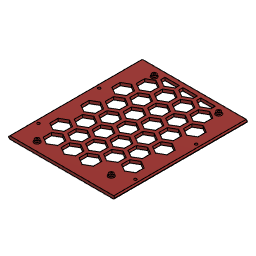
MCU Tray - BTT Manta M8P (Autodesk Fusion 360 design; units mm, degrees)
Autodesk Fusion 360 part; units mm, degrees
note: some values were not read from the file. Chosen so that the rebuilt part matches the saved one: a direction.
imported_body "Derived Base Feature2" makes body 1
imported_body "Derived Base Feature1" makes body 2
sketch "Base Profile" plane through (0, 0, 0) normal (0, 1, 0) x (1, 0, 0)
  line L0 (72.5, 2) -> (-72.5, 2)
  line L1 (-72.5, 2) -> (-72.5, -2) construction
  line L2 (-72.5, -2) -> (72.5, -2)
  line L3 (72.5, -2) -> (72.5, 2) construction
  line L4 (72.5, 2) -> (-72.5, -2) construction
  line L5 (-72.5, 2) -> (72.5, -2) construction
  line L6 (-72.5, 0) -> (-74.3, 0) construction
  line L7 (-72.5, -2) -> (-74.3, -0.2)
  line L8 (-74.3, 0.2) -> (-72.5, 2)
  line L9 (-74.3, -0.2) -> (-74.3, 0)
  line L10 (-74.3, 0) -> (-74.3, 0.2)
  line L11 (0, 0) -> (0, -2) construction
  line L12 (72.5, -2) -> (74.3, -0.2)
  line L13 (74.3, -0.2) -> (74.3, 0)
  line L14 (74.3, 0) -> (74.3, 0.2)
  line L15 (74.3, 0.2) -> (72.5, 2)
  dimension "d1" = 145
  dimension "d2" = 4
  dimension "d3" = 0.2
  constraint horizontal L0
  constraint perpendicular L0 L1
  constraint parallel L0 L2
  constraint parallel L1 L3
  constraint coincident L4 L11.start
  constraint coincident L5 L11.start
  constraint coincident L11.start origin
  constraint midpoint L1 L6.start
  constraint perpendicular L1 L6
  constraint coincident L5 L0.end
  constraint coincident L0 L1.start
  constraint perpendicular L6 L9
  constraint perpendicular L6 L10
  constraint midpoint L2 L11.end
  constraint symmetric L1.end L11 L2.end
  constraint symmetric L0.end L11 L0.start
  constraint symmetric L7.end L11 L12.end
  constraint symmetric L6.end L11 L13.end
  constraint symmetric L8.start L11 L14.end
  measures "d1" distance of L1.end L2.end
  measures "d2" distance of L0.end L1.end
  measures "d3" distance of L7.end L6.end
extrude "Extrude1" add sketch "Base Profile" along normal blind 190 and the other way blind 15 separate body makes body 3
sketch "M3 Mount Holes" plane through (0, 0, 2) normal (0, 0, 1) x (-1, 0, 0)
  line L0 (72.5, 15) -> (-72.5, 15)
  line L1 (-72.5, 15) -> (-72.5, -190)
  line L2 (-72.5, -190) -> (72.5, -190)
  line L3 (72.5, -190) -> (72.5, 15)
  line L4 (0, 0) -> (0, -28.0831) construction
  circle A0 centre (-67.6414, -20) radius 1.8
  line L5 (72.6414, -59.8458) -> (72.6414, 0.0002) construction
  circle A1 centre (67.6414, -20) radius 1.8
  line L6 (72.5, -190) -> (72.5, 15)
  line L7 (72.6414, 0.0002) -> (78.5, 0.0002)
  line L8 (67.6414, -20) -> (72.6414, -20) construction
  line L9 (72.6414, -20) -> (72.6414, 0.0002) construction
  line L10 (67.6414, -20) -> (67.6414, -105) construction
  circle A2 centre (67.6414, -105) radius 1.8
  circle A3 centre (-67.6414, -105) radius 1.8
  dimension "d16" = 3.6
  dimension "d17" = 85
  dimension "d18" = 3.6
  dimension "d42" = 5
  dimension "d43" = 35
  constraint coincident L4.start origin
  constraint vertical L4
  constraint symmetric L4 A0 A1
  constraint horizontal L8
  constraint vertical L9
  constraint coincident L5.end L7.start
  constraint coincident A1.centre L8.start
  constraint perpendicular L8 L10
  constraint coincident L10.end A2.centre
  constraint symmetric L4 A2 A3
  measures "d16" diameter of A1
  measures "d17" distance of A1.centre L10.end
  measures "d18" diameter of A2
  measures "d42" distance of A1.centre L8.end
  measures "d43" distance of L0 A1.centre
sketch "M4 Mount Holes" plane through (0, 0, 2) normal (0, 0, 1) x (-1, 0, 0)
  line L0 (-72.5, 15) -> (-72.5, -190)
  line L1 (-72.5, -190) -> (72.5, -190)
  line L2 (72.5, -190) -> (72.5, 15)
  line L3 (72.5, 15) -> (-72.5, 15)
  circle A0 centre (-67.6414, -20) radius 1.8 construction
  circle A1 centre (-67.6414, -20) radius 2.3
  line L4 (-67.6414, -20) -> (-67.6414, -105) construction
  circle A2 centre (-67.6414, -105) radius 2.3
  line L5 (0, 0) -> (0, -39.5368) construction
  circle A3 centre (67.6414, -105) radius 2.3
  circle A4 centre (67.6414, -20) radius 2.3
  dimension "d37" = 4.6
  dimension "d38" = 85
  dimension "d39" = 4.6
  constraint concentric A0 A1
  constraint coincident A0.centre A1.centre
  constraint parallel L0 L4
  constraint coincident L4.end A2.centre
  constraint coincident L5.start origin
  constraint vertical L5
  constraint symmetric A1 L5 A4
  constraint symmetric A2 L5 A3
  measures "d37" diameter of A1
  measures "d38" distance of A0.centre L4.end
  measures "d39" diameter of A2
extrude "Extrude2" cut sketch "M3 Mount Holes" against normal up to surface (4 mm away) contours A0 | A1 | A2 | A3 bodies 3
extrude "Extrude5" [suppressed]
extrude "Extrude3" cut 1 faces at (24.1667, 190, 0.6667) along direction (0, -1, 0) blind 40.154 on bodies 3 bodies 3
delete_body "RemoveBody1" bodies 2
delete_body "RemoveBody2" bodies 1
move_face "OffsetFaces2" offset 20 1 faces at (24.1667, 149.846, 0.6667) on bodies 3
sketch "Vent Holes" plane through (0, 0, 2) normal (0, 0, 1) x (-1, 0, 0)
  line L0 (-72.5, -169.846) -> (72.5, -169.846)
  line L1 (72.5, -169.846) -> (72.5, 15)
  line L2 (72.5, 15) -> (-72.5, 15)
  line L3 (-72.5, 15) -> (-72.5, -169.846)
  line L4 (0, 15) -> (0, -169.846) construction
  line L5 (10, -71.6495) -> (0, -65.876)
  line L6 (0, -65.876) -> (-10, -71.6495)
  line L7 (-10, -71.6495) -> (-10, -83.1965)
  line L8 (-10, -83.1965) -> (0, -88.97)
  line L9 (0, -88.97) -> (10, -83.1965)
  line L10 (10, -83.1965) -> (10, -71.6495)
  line L11 (0, -77.423) -> (5, -86.0833) construction
  line L12 (0, -77.423) -> (-5, -86.0833) construction
  line L13 (-15, -28.3482) -> (-25, -22.5747)
  line L14 (-25, -22.5747) -> (-35, -28.3482)
  line L15 (-35, -28.3482) -> (-35, -39.8952)
  line L16 (-35, -39.8952) -> (-25, -45.6687)
  line L17 (-25, -45.6687) -> (-15, -39.8952)
  line L18 (-15, -39.8952) -> (-15, -28.3482)
  line L19 (-27.5, -6.6976) -> (-37.5, -0.9241)
  line L20 (-37.5, -0.9241) -> (-47.5, -6.6976)
  line L21 (-47.5, -6.6976) -> (-47.5, -18.2446)
  line L22 (-47.5, -18.2446) -> (-37.5, -24.0181)
  line L23 (-37.5, -24.0181) -> (-27.5, -18.2446)
  line L24 (-27.5, -18.2446) -> (-27.5, -6.6976)
  line L25 (-2.5, -49.9989) -> (-12.5, -44.2254)
  line L26 (-12.5, -44.2254) -> (-22.5, -49.9989)
  line L27 (-22.5, -49.9989) -> (-22.5, -61.5459)
  line L28 (-22.5, -61.5459) -> (-12.5, -67.3194)
  line L29 (-12.5, -67.3194) -> (-2.5, -61.5459)
  line L30 (-2.5, -61.5459) -> (-2.5, -49.9989)
  line L31 (22.5, -93.3001) -> (12.5, -87.5266)
  line L32 (12.5, -87.5266) -> (2.5, -93.3001)
  line L33 (2.5, -93.3001) -> (2.5, -104.8471)
  line L34 (2.5, -104.8471) -> (12.5, -110.6206)
  line L35 (12.5, -110.6206) -> (22.5, -104.8471)
  line L36 (22.5, -104.8471) -> (22.5, -93.3001)
  line L37 (35, -114.9508) -> (25, -109.1773)
  line L38 (25, -109.1773) -> (15, -114.9508)
  line L39 (15, -114.9508) -> (15, -126.4978)
  line L40 (15, -126.4978) -> (25, -132.2713)
  line L41 (25, -132.2713) -> (35, -126.4978)
  line L42 (35, -126.4978) -> (35, -114.9508)
  line L43 (47.5, -136.6014) -> (37.5, -130.8279)
  line L44 (37.5, -130.8279) -> (27.5, -136.6014)
  line L45 (27.5, -136.6014) -> (27.5, -148.1484)
  line L46 (27.5, -148.1484) -> (37.5, -153.9219)
  line L47 (37.5, -153.9219) -> (47.5, -148.1484)
  line L48 (47.5, -148.1484) -> (47.5, -136.6014)
  line L49 (12.5, -67.3194) -> (22.5, -61.5459)
  line L50 (22.5, -61.5459) -> (22.5, -49.9989)
  line L51 (22.5, -49.9989) -> (12.5, -44.2254)
  line L52 (12.5, -44.2254) -> (2.5, -49.9989)
  line L53 (2.5, -61.5459) -> (12.5, -67.3194)
  line L54 (2.5, -49.9989) -> (2.5, -61.5459)
  line L55 (-15, -71.6495) -> (-25, -65.876)
  line L56 (-25, -65.876) -> (-35, -71.6495)
  line L57 (-35, -71.6495) -> (-35, -83.1965)
  line L58 (-35, -83.1965) -> (-25, -88.97)
  line L59 (-15, -83.1965) -> (-15, -71.6495)
  line L60 (-25, -88.97) -> (-15, -83.1965)
  line L61 (-2.5, -6.6976) -> (-12.5, -0.9241)
  line L62 (-12.5, -0.9241) -> (-22.5, -6.6976)
  line L63 (-22.5, -6.6976) -> (-22.5, -18.2446)
  line L64 (-22.5, -18.2446) -> (-12.5, -24.0181)
  line L65 (-12.5, -24.0181) -> (-2.5, -18.2446)
  line L66 (-2.5, -18.2446) -> (-2.5, -6.6976)
  line L67 (-40, -28.3482) -> (-50, -22.5747)
  line L68 (-50, -22.5747) -> (-60, -28.3482)
  line L69 (-60, -28.3482) -> (-60, -39.8952)
  line L70 (-60, -39.8952) -> (-50, -45.6687)
  line L71 (-40, -39.8952) -> (-40, -28.3482)
  line L72 (-50, -45.6687) -> (-40, -39.8952)
  line L73 (10, -28.3482) -> (0, -22.5747)
  line L74 (0, -22.5747) -> (-10, -28.3482)
  line L75 (-10, -28.3482) -> (-10, -39.8952)
  line L76 (-10, -39.8952) -> (0, -45.6687)
  line L77 (0, -45.6687) -> (10, -39.8952)
  line L78 (10, -39.8952) -> (10, -28.3482)
  line L79 (-27.5, -49.9989) -> (-37.5, -44.2254)
  line L80 (-37.5, -44.2254) -> (-47.5, -49.9989)
  line L81 (-47.5, -49.9989) -> (-47.5, -61.5459)
  line L82 (-47.5, -61.5459) -> (-37.5, -67.3194)
  line L83 (-27.5, -61.5459) -> (-27.5, -49.9989)
  line L84 (-37.5, -67.3194) -> (-27.5, -61.5459)
  line L85 (35, -71.6495) -> (25, -65.876)
  line L86 (25, -65.876) -> (15, -71.6495)
  line L87 (15, -71.6495) -> (15, -83.1965)
  line L88 (15, -83.1965) -> (25, -88.97)
  line L89 (25, -88.97) -> (35, -83.1965)
  line L90 (35, -83.1965) -> (35, -71.6495)
  line L91 (-2.5, -93.3001) -> (-12.5, -87.5266)
  line L92 (-12.5, -87.5266) -> (-22.5, -93.3001)
  line L93 (-22.5, -93.3001) -> (-22.5, -104.8471)
  line L94 (-22.5, -104.8471) -> (-12.5, -110.6206)
  line L95 (-2.5, -104.8471) -> (-2.5, -93.3001)
  line L96 (-12.5, -110.6206) -> (-2.5, -104.8471)
  line L97 (47.5, -93.3001) -> (37.5, -87.5266)
  line L98 (37.5, -87.5266) -> (27.5, -93.3001)
  line L99 (27.5, -93.3001) -> (27.5, -104.8471)
  line L100 (27.5, -104.8471) -> (37.5, -110.6206)
  line L101 (37.5, -110.6206) -> (47.5, -104.8471)
  line L102 (47.5, -104.8471) -> (47.5, -93.3001)
  line L103 (10, -114.9508) -> (0, -109.1773)
  line L104 (0, -109.1773) -> (-10, -114.9508)
  line L105 (-10, -114.9508) -> (-10, -126.4978)
  line L106 (-10, -126.4978) -> (0, -132.2713)
  line L107 (10, -126.4978) -> (10, -114.9508)
  line L108 (0, -132.2713) -> (10, -126.4978)
  line L109 (60, -114.9508) -> (50, -109.1773)
  line L110 (50, -109.1773) -> (40, -114.9508)
  line L111 (40, -114.9508) -> (40, -126.4978)
  line L112 (40, -126.4978) -> (50, -132.2713)
  line L113 (50, -132.2713) -> (60, -126.4978)
  line L114 (60, -126.4978) -> (60, -114.9508)
  line L115 (22.5, -136.6014) -> (12.5, -130.8279)
  line L116 (12.5, -130.8279) -> (2.5, -136.6014)
  line L117 (2.5, -136.6014) -> (2.5, -148.1484)
  line L118 (2.5, -148.1484) -> (12.5, -153.9219)
  line L119 (22.5, -148.1484) -> (22.5, -136.6014)
  line L120 (12.5, -153.9219) -> (22.5, -148.1484)
  line L121 (-47.5, -55.7724) -> (-60, -55.7724) construction
  line L122 (-40, -71.6495) -> (-40, -83.1965)
  line L123 (-40, -83.1965) -> (-50, -88.97)
  line L124 (-50, -88.97) -> (-60, -83.1965)
  line L125 (-60, -83.1965) -> (-60, -71.6495)
  line L126 (-60, -71.6495) -> (-50, -65.876)
  line L127 (-50, -65.876) -> (-40, -71.6495)
  line L128 (47.5, -99.0736) -> (60, -99.0736) construction
  line L129 (40, -83.1965) -> (40, -71.6495)
  line L130 (40, -71.6495) -> (50, -65.876)
  line L131 (50, -65.876) -> (60, -71.6495)
  line L132 (60, -71.6495) -> (60, -83.1965)
  line L133 (60, -83.1965) -> (50, -88.97)
  line L134 (50, -88.97) -> (40, -83.1965)
  line L135 (-47.5, -104.8471) -> (-47.5, -93.3001)
  line L136 (-47.5, -93.3001) -> (-37.5, -87.5266)
  line L137 (-37.5, -87.5266) -> (-27.5, -93.3001)
  line L138 (-27.5, -93.3001) -> (-27.5, -104.8471)
  line L139 (-27.5, -104.8471) -> (-37.5, -110.6206)
  line L140 (-37.5, -110.6206) -> (-47.5, -104.8471)
  line L141 (-60, -126.4978) -> (-60, -114.9508)
  line L142 (-60, -114.9508) -> (-50, -109.1773)
  line L143 (-50, -109.1773) -> (-40, -114.9508)
  line L144 (-40, -114.9508) -> (-40, -126.4978)
  line L145 (-50, -132.2713) -> (-60, -126.4978)
  line L146 (-40, -126.4978) -> (-50, -132.2713)
  line L147 (-27.5, -136.6014) -> (-27.5, -148.1484)
  line L148 (-27.5, -148.1484) -> (-37.5, -153.9219)
  line L149 (-37.5, -153.9219) -> (-47.5, -148.1484)
  line L150 (-47.5, -148.1484) -> (-47.5, -136.6014)
  line L151 (-37.5, -130.8279) -> (-27.5, -136.6014)
  line L152 (-47.5, -136.6014) -> (-37.5, -130.8279)
  line L153 (-35, -114.9508) -> (-25, -109.1773)
  line L154 (-25, -109.1773) -> (-15, -114.9508)
  line L155 (-15, -114.9508) -> (-15, -126.4978)
  line L156 (-15, -126.4978) -> (-25, -132.2713)
  line L157 (-35, -126.4978) -> (-35, -114.9508)
  line L158 (-25, -132.2713) -> (-35, -126.4978)
  line L159 (27.5, -49.9989) -> (37.5, -44.2254)
  line L160 (37.5, -44.2254) -> (47.5, -49.9989)
  line L161 (47.5, -49.9989) -> (47.5, -61.5459)
  line L162 (47.5, -61.5459) -> (37.5, -67.3194)
  line L163 (27.5, -61.5459) -> (27.5, -49.9989)
  line L164 (37.5, -67.3194) -> (27.5, -61.5459)
  line L165 (15, -28.3482) -> (25, -22.5747)
  line L166 (25, -22.5747) -> (35, -28.3482)
  line L167 (35, -28.3482) -> (35, -39.8952)
  line L168 (35, -39.8952) -> (25, -45.6687)
  line L169 (15, -39.8952) -> (15, -28.3482)
  line L170 (25, -45.6687) -> (15, -39.8952)
  line L171 (27.5, -6.6976) -> (37.5, -0.9241)
  line L172 (37.5, -0.9241) -> (47.5, -6.6976)
  line L173 (47.5, -6.6976) -> (47.5, -18.2446)
  line L174 (47.5, -18.2446) -> (37.5, -24.0181)
  line L175 (27.5, -18.2446) -> (27.5, -6.6976)
  line L176 (37.5, -24.0181) -> (27.5, -18.2446)
  line L177 (40, -28.3482) -> (50, -22.5747)
  line L178 (50, -22.5747) -> (60, -28.3482)
  line L179 (60, -28.3482) -> (60, -39.8952)
  line L180 (60, -39.8952) -> (50, -45.6687)
  line L181 (40, -39.8952) -> (40, -28.3482)
  line L182 (50, -45.6687) -> (40, -39.8952)
  line L183 (22.5, -6.6976) -> (22.5, -18.2446)
  line L184 (22.5, -18.2446) -> (12.5, -24.0181)
  line L185 (12.5, -24.0181) -> (2.5, -18.2446)
  line L186 (2.5, -18.2446) -> (2.5, -6.6976)
  line L187 (12.5, -0.9241) -> (22.5, -6.6976)
  line L188 (2.5, -6.6976) -> (12.5, -0.9241)
  line L189 (-2.5, -136.6014) -> (-2.5, -148.1484)
  line L190 (-2.5, -148.1484) -> (-12.5, -153.9219)
  line L191 (-12.5, -153.9219) -> (-22.5, -148.1484)
  line L192 (-22.5, -148.1484) -> (-22.5, -136.6014)
  line L193 (-12.5, -130.8279) -> (-2.5, -136.6014)
  line L194 (-22.5, -136.6014) -> (-12.5, -130.8279)
  circle A0 centre (-67.6414, -105) radius 1.8
  circle A1 centre (-67.6414, -20) radius 1.8
  circle A2 centre (67.6414, -105) radius 1.8
  circle A3 centre (67.6414, -20) radius 1.8
  line L195 (-47.5, -142.3749) -> (-60, -142.3749) construction
  line L196 (-15, -164.0255) -> (-15, -158.252)
  line L197 (-15, -158.252) -> (-25, -152.4785)
  line L198 (-35, -158.252) -> (-35, -164.0255)
  line L199 (-25, -152.4785) -> (-35, -158.252)
  line L200 (10, -158.252) -> (10, -164.0255)
  line L201 (-10, -164.0255) -> (-10, -158.252)
  line L202 (0, -152.4785) -> (10, -158.252)
  line L203 (-10, -158.252) -> (0, -152.4785)
  line L204 (35, -158.252) -> (35, -164.0255)
  line L205 (15, -164.0255) -> (15, -158.252)
  line L206 (25, -152.4785) -> (35, -158.252)
  line L207 (15, -158.252) -> (25, -152.4785)
  line L208 (-15, -164.0255) -> (-35, -164.0255)
  line L209 (35, -164.0255) -> (15, -164.0255)
  line L210 (10, -164.0255) -> (-10, -164.0255)
  point P0 (0, -77.423)
  dimension "d19" = 10
  dimension "d22" = 25
  dimension "d23" = 50
  dimension "d29" = 360
  dimension "d32" = 25
  dimension "d33" = 0
  constraint midpoint L2 L4.start
  constraint midpoint L0 L4.end
  constraint midpoint L4 P0
  constraint coincident P0 L11.start
  constraint midpoint L9 L11.end
  constraint midpoint L8 L12.end
  constraint midpoint L81 L121.start
  constraint perpendicular L81 L121
  constraint symmetric L67.start L121 L122.end
  constraint symmetric L67.end L121 L123.end
  constraint symmetric L68.end L121 L124.end
  constraint symmetric L69.end L121 L125.end
  constraint symmetric L70.end L121 L126.end
  constraint symmetric L71.start L121 L122.start
  constraint midpoint L102 L128.start
  constraint perpendicular L102 L128
  constraint symmetric L109.start L128 L132.end
  constraint symmetric L109.end L128 L133.end
  constraint symmetric L110.end L128 L129.start
  constraint symmetric L111.end L128 L129.end
  constraint symmetric L112.end L128 L130.end
  constraint symmetric L113.end L128 L131.end
  constraint symmetric L4 L13.start L165.start
  constraint symmetric L4 L13.end L165.end
  constraint symmetric L4 L14.end L166.end
  constraint symmetric L4 L15.end L167.end
  constraint symmetric L4 L16.end L168.end
  constraint symmetric L4 L17.end L169.start
  constraint symmetric L4 L19.start L171.start
  constraint symmetric L4 L19.end L171.end
  constraint symmetric L4 L20.end L172.end
  constraint symmetric L4 L21.end L173.end
  constraint symmetric L4 L22.end L174.end
  constraint symmetric L4 L23.end L175.start
  constraint symmetric L4 L37.start L153.start
  constraint symmetric L4 L37.end L153.end
  constraint symmetric L4 L38.end L154.end
  constraint symmetric L4 L39.end L155.end
  constraint symmetric L4 L40.end L156.end
  constraint symmetric L4 L41.end L157.start
  constraint symmetric L4 L43.start L150.end
  constraint symmetric L4 L43.end L151.start
  constraint symmetric L4 L44.end L147.start
  constraint symmetric L4 L45.end L147.end
  constraint symmetric L4 L46.end L148.end
  constraint symmetric L4 L47.end L149.end
  constraint symmetric L4 L61.start L186.end
  constraint symmetric L4 L61.end L187.start
  constraint symmetric L4 L62.end L183.start
  constraint symmetric L4 L63.end L183.end
  constraint symmetric L4 L64.end L184.end
  constraint symmetric L4 L65.end L185.end
  constraint symmetric L4 L67.start L177.start
  constraint symmetric L4 L67.end L177.end
  constraint symmetric L4 L68.end L178.end
  constraint symmetric L4 L69.end L179.end
  constraint symmetric L4 L70.end L180.end
  constraint symmetric L4 L71.start L181.start
  constraint symmetric L4 L79.start L159.start
  constraint symmetric L4 L79.end L159.end
  constraint symmetric L4 L80.end L160.end
  constraint symmetric L4 L81.end L161.end
  constraint symmetric L4 L82.end L162.end
  constraint symmetric L4 L83.start L163.start
  constraint symmetric L4 L97.start L135.end
  constraint symmetric L4 L97.end L136.end
  constraint symmetric L4 L98.end L137.end
  constraint symmetric L4 L99.end L138.end
  constraint symmetric L4 L100.end L139.end
  constraint symmetric L4 L101.end L135.start
  constraint symmetric L4 L109.start L141.end
  constraint symmetric L4 L109.end L142.end
  constraint symmetric L4 L110.end L143.end
  constraint symmetric L4 L111.end L144.end
  constraint symmetric L4 L112.end L145.start
  constraint symmetric L4 L113.end L141.start
  constraint symmetric L4 L115.start L192.end
  constraint symmetric L4 L115.end L193.start
  constraint symmetric L4 L116.end L189.start
  constraint symmetric L4 L117.end L189.end
  constraint symmetric L4 L118.end L190.end
  constraint symmetric L4 L119.start L191.end
  constraint midpoint L150 L195.start
  constraint perpendicular L150 L195
  constraint symmetric L39.end L195 L205.end
  constraint symmetric L40.end L195 L206.start
  constraint symmetric L41.end L195 L204.start
  constraint symmetric L105.end L195 L201.end
  constraint symmetric L106.end L195 L202.start
  constraint symmetric L107.start L195 L200.start
  constraint symmetric L155.end L195 L196.end
  constraint symmetric L156.end L195 L197.end
  constraint symmetric L157.start L195 L198.start
  constraint coincident L200.end L209
  constraint collinear L208 L209
  constraint collinear L209 L210
  measures "d19" distance of P0 L10
sketch "Mounting Holes" plane through (0, 0, 2) normal (0, 0, 1) x (-1, 0, 0)
  line L0 (-72.5, -169.846) -> (72.5, -169.846)
  line L1 (72.5, -169.846) -> (72.5, 15)
  line L2 (72.5, 15) -> (-72.5, 15)
  line L3 (-72.5, 15) -> (-72.5, -169.846)
  circle A0 centre (-67.6414, -105) radius 1.8
  circle A1 centre (-67.6414, -20) radius 1.8
  circle A2 centre (67.6414, -105) radius 1.8
  circle A3 centre (67.6414, -20) radius 1.8
  line L4 (0, 15) -> (0, -169.846) construction
  line L5 (51.3715, -162.3894) -> (-51.3715, -162.3894) construction
  line L6 (-51.3715, -162.3894) -> (-51.3715, 7.5366) construction
  line L7 (-51.3715, 7.5366) -> (51.3715, 7.5366) construction
  line L8 (51.3715, 7.5366) -> (51.3715, -162.3894) construction
  line L9 (51.3715, -77.4264) -> (-51.3715, -77.4264) construction
  line L10 (-51.3715, -162.3894) -> (-46.6285, -162.3894) construction
  line L11 (-46.6285, -162.3894) -> (-46.6285, -157.3894) construction
  circle A4 centre (-46.6285, -157.3894) radius 1.4
  circle A5 centre (-46.6285, -157.3894) radius 3
  line L12 (-46.6285, -157.3894) -> (-46.6285, -7.3894) construction
  circle A6 centre (-46.6285, -7.3894) radius 1.4
  circle A7 centre (-46.6285, -7.3894) radius 3
  line L13 (-46.6285, -157.3894) -> (43.3715, -157.3894) construction
  circle A8 centre (43.3715, -157.3894) radius 1.4
  circle A9 centre (43.3715, -157.3894) radius 3
  circle A10 centre (46.3715, 3.0589) radius 1.4
  circle A11 centre (46.3715, 3.0589) radius 3
  line L14 (46.3715, 3.0589) -> (51.3715, 3.0589) construction
  point P0 (0, -77.423)
  dimension "d45" = 102.743
  dimension "d46" = 169.926
  dimension "d48" = 5
  dimension "d49" = 2.8
  dimension "d50" = 1.6
  dimension "d51" = 150
  dimension "d52" = 2.8
  dimension "d53" = 1.6
  dimension "d54" = 90
  dimension "d55" = 2.8
  dimension "d56" = 1.6
  dimension "d58" = 2.8
  dimension "d59" = 1.6
  dimension "d68" = 5
  dimension "d69" = 8
  dimension "d70" = 4.743
  constraint midpoint L2 L4.start
  constraint midpoint L0 L4.end
  constraint horizontal L5
  constraint perpendicular L5 L6
  constraint parallel L5 L7
  constraint parallel L6 L8
  constraint midpoint L4 P0
  constraint midpoint L8 L9.start
  constraint midpoint L6 L9.end
  constraint perpendicular L6 L10
  constraint perpendicular L10 L11
  constraint coincident L11.end A4.centre
  constraint parallel L11 L12
  constraint coincident L12.end A6.centre
  constraint perpendicular L11 L13
  constraint coincident L13.end A8.centre
  constraint coincident A10.centre A11.centre
  constraint perpendicular L8 L14
  constraint coincident L8 L14.end
  measures "d45" distance of L6.end L7.end
  measures "d46" distance of L5.start L7.end
  measures "d48" distance of L10.end L11.end
  measures "d49" diameter of A4
  measures "d51" distance of L11.end L12.end
  measures "d52" diameter of A6
  measures "d54" distance of L11.end L13.end
  measures "d55" diameter of A8
  measures "d58" diameter of A10
  measures "d68" distance of A10.centre L14.end
  measures "d69" distance of L8 L13.end
  measures "d70" distance of L6 L11
extrude "Extrude4" cut sketch "Vent Holes" against normal blind 8 contours L5 L6 L7 L8 L9 L10 | L13 L14 L15 L16 L17 L18 | L25 L26 L27 L28 L29 L30 | L31 L32 L33 L34 L35 L36 | L37 L38 L39 L40 L41 L42 | L43 L44 L45 L46 L47 L48 | L49 L50 L51 L52 L53 L54 | L55 L56 L57 L58 L59 L60 | L61 L62 L63 L64 L65 L66 | L67 L68 L69 L70 L71 L72 | L73 L74 L75 L76 L77 L78 | L79 L80 L81 L82 L83 L84 | L85 L86 L87 L88 L89 L90 | L91 L92 L93 L94 L95 L96 | L97 L98 L99 L100 L101 L102 | L103 L104 L105 L106 L107 L108 | L109 L110 L111 L112 L113 L114 | L115 L116 L117 L118 L119 L120 | L122 L123 L124 L125 L126 L127 | L129 L130 L131 L132 L133 L134 | L135 L136 L137 L138 L139 L140 | L141 L142 L143 L144 L145 L146 | L147 L148 L149 L150 L151 L152 | L153 L154 L155 L156 L157 L158 | L159 L160 L161 L162 L163 L164 | L165 L166 L167 L168 L169 L170 | L171 L172 L173 L174 L175 L176 | L177 L178 L179 L180 L181 L182 | L183 L184 L185 L186 L187 L188 | L189 L190 L191 L192 L193 L194 | L196 L197 L198 L199 L208 | L200 L201 L202 L203 L210 | L204 L205 L206 L207 L209 bodies 3
extrude "Extrude7" cut sketch "Mounting Holes" against normal blind 4 contours A4 | A6 | A8 | A10 bodies 3
extrude "Extrude6" add sketch "Mounting Holes" along normal blind 3 contours A5 | A7 | A9 | A11 bodies 3
fillet "Fillet1" radius 1 4 edges at (49.4255, 156.3045, 2) (-40.5745, 156.3045, 2) (49.4255, 6.3045, 2) (-43.5745, -4.1437, 2) on bodies 3
equation "d18 = d16"
named bodies: "Body1 (Context1)", "Body1 (Context2)"
